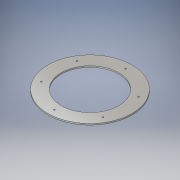
# Autodesk Inventor part: Turret Gear
Saved by Autodesk Inventor 2016 (Build 200138000, 138)
## iProperties
Created: 2018-06-21
Part Number: Turret Gear
Material: Generic
Document SubType Name: Modeling
Designer: Kade
Density: 1 g/cm^3
Appearance: Aluminum - Dark
Author: Kade
Autodesk Inventor part; units mm, degrees
ref_plane "YZ Plane" through (0, 0, 0) normal (1, 0, 0) x (0, 1, 0)
ref_plane "XZ Plane" through (0, 0, 0) normal (0, 1, 0) x (-1, 0, 0)
ref_plane "XY Plane" through (0, 0, 0) normal (0, 0, 1) x (1, 0, 0)
sketch "Sketch1" plane through (0, 0, 0) normal (0, 1, 0) x (-1, 0, 0)
  circle A0 centre (0, 0) radius 190.5
  circle A1 centre (0, 0) radius 130.175
  circle A2 centre (0, -161.3591) radius 3.2258
  circle A3 centre (139.741, -80.6795) radius 3.2258
  circle A4 centre (139.741, 80.6795) radius 3.2258
  circle A5 centre (0, 161.3591) radius 3.2258
  circle A6 centre (-139.741, 80.6795) radius 3.2258
  circle A7 centre (-139.741, -80.6795) radius 3.2258
  dimension "d0" = 381
  dimension "d1" = 260.35
  dimension "d4" = 6.4516
  dimension "d7" = 360
  constraints: 8 centre point, 2 coincident, 13 other
  measures "d0" diameter of A0
  measures "d1" diameter of A1
  measures "d4" diameter of A2
extrude "Extrusion3" add sketch "Sketch1" along normal blind 6.35
body "Solid3"
